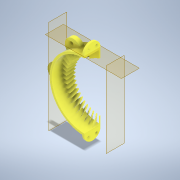
# Autodesk Inventor part: HalfShell.48.3.0
Saved by Autodesk Inventor 2021.2 (Build 252289000, 289)
## iProperties
Created: 2021-03-12
Part Number: HalfShell.48.3.0
Material: Generic
Document SubType Name: Modeling
Designer: Ryan
Density: 1 g/cm^3
Appearance: Smooth - Yellow
Author: Ryan
## iProperties of the stored document _3DPrint.ipt
Created: 2021-05-17
Part Number: _3DPrint
Material: Generic
Document SubType Name: Modeling
Designer: Ryan
Density: 1 g/cm^3
Appearance: Default
Author: Ryan
Autodesk Inventor part; units mm, degrees
ref_plane "XY Plane" through (0, 0, 0) normal (0, 0, 1) x (1, 0, 0)
sketch "Sketch1" plane through (0, 0, 0) normal (0, 0, 1) x (1, 0, 0)
  circle A0 centre (0, 0) radius 50.8
  circle A1 centre (0, 0) radius 53.975
  dimension "d0" = 101.6
  dimension "d1" = 107.95
  constraints: 2 centre point, 2 coincident
  measures "d0" diameter of A0
  measures "d1" diameter of A1
extrude "Extrusion1" add sketch "Sketch1" along normal blind 25.4
ref_plane "Work Plane1" through (35.56, 0, 0) normal (1, 0, 0) x (0, 1, 0)
ref_plane "Work Plane2" through (0, 53.975, 0) normal (0, 1, 0) x (-1, 0, 0)
sketch "Sketch3" plane through (0, 53.975, 0) normal (0, 1, 0) x (-1, 0, 0)
  line L0 (53.975, 0) -> (-53.975, 0) projected
  line L1 (3.175, 25.4) -> (-3.175, 25.4)
  line L2 (-3.175, 25.4) -> (-3.175, 0)
  line L3 (-3.175, 0) -> (3.175, 0)
  line L4 (3.175, 0) -> (3.175, 25.4)
  line L5 (3.175, 25.4) -> (-3.175, 0) construction
  line L6 (-3.175, 25.4) -> (3.175, 0) construction
  line L7 (53.975, 25.4) -> (-53.975, 25.4) projected
  point P0 (0, 0)
  point P1 (0, 12.7)
  point P2 (3.175, 0)
  dimension "d11" = 6.35
  dimension "d12" = 0
  constraints: 12 end point, 2 midpoint, 2 parallel, 1 horizontal, 1 perpendicular, 1 point on line
  measures "d11" distance of L3.end L2.end
  measures "d12" distance between parallel lines of L7 L1
extrude "Extrusion3" add sketch "Sketch3" along normal blind 12.7
fillet "Fillet1" radius 12.7 2 edges at (0, 66.675, 25.4) (0, 66.675, 0)
sketch "Sketch4" plane through (3.175, 53.975, 25.4) normal (1, 0, 0) x (0, 0, -1)
  circle A0 centre (6.35, 5.08) radius 1.5875
  line L0 (-5.08, 0) -> (30.48, 0) projected
  line L1 (0, 0) -> (0, -107.95) projected
  circle A1 centre (19.05, 5.08) radius 1.5875
  line L2 (25.4, 0) -> (25.4, -107.95) projected
  point P0 (25.4, -53.975)
  dimension "d16" = 3.175
  dimension "d17" = 5.08
  dimension "d40" = 6.35
  dimension "d41" = 3.175
  dimension "d42" = 6.35
  dimension "d43" = 5.08
  constraints: 2 centre point
  measures "d16" diameter of A0
  measures "d17" distance from line of L0 A0.centre
  measures "d40" horizontal distance of A0.centre L1.start
  measures "d41" diameter of A1
  measures "d42" horizontal distance of L2.start A1.centre
  measures "d43" distance from line of L0 A1.centre
extrude "Extrusion4" cut sketch "Sketch4" against normal blind 12.7
pattern_circular "Circular Pattern2" count 2 over 360 about axis through (0, 0, 0) along (0, 0, 1) of "Extrusion4", "Fillet1", "Extrusion3"
ref_plane "Work Plane3" through (-53.975, 0, 0) normal (1, 0, 0) x (0, 1, 0)
sketch "Sketch5" plane through (-53.975, 0, 0) normal (1, 0, 0) x (0, 1, 0)
  line L0 (-12.7, 9.525) -> (12.7, 9.525)
  line L1 (12.7, 9.525) -> (12.7, 15.875)
  line L2 (12.7, 15.875) -> (-12.7, 15.875)
  line L3 (-12.7, 15.875) -> (-12.7, 9.525)
  line L4 (-12.7, 9.525) -> (12.7, 15.875) construction
  line L5 (12.7, 9.525) -> (-12.7, 15.875) construction
  point P0 (0, 0)
  point P1 (0, 12.7)
  dimension "d24" = 25.4
  dimension "d25" = 6.35
  dimension "d26" = 12.7
  dimension "d27" = 0
  constraints: 12 end point, 2 midpoint, 2 parallel, 1 horizontal, 1 perpendicular
  measures "d24" distance of L2.end L1.end
  measures "d25" distance of L1.end L0.end
  measures "d26" distance of point (0, 12.7) point (0, 0)
  measures "d27" horizontal distance of point (0, 12.7) point (0, 0)
extrude "Extrusion5" add sketch "Sketch5" along normal blind 2.54
sketch "Sketch6" plane through (-53.975, 0, 0) normal (-1, 0, 0) x (0, 0, 1)
  line L0 (15.875, 0) -> (15.875, -12.7) projected
  line L1 (9.525, 12.7) -> (15.875, 12.7)
  line L2 (15.875, 12.7) -> (15.875, -12.7)
  line L3 (15.875, -12.7) -> (9.525, -12.7)
  line L4 (9.525, -12.7) -> (9.525, 12.7)
  line L5 (9.525, 12.7) -> (15.875, -12.7) construction
  line L6 (15.875, 12.7) -> (9.525, -12.7) construction
  point P0 (0, 0)
  point P1 (12.7, 0)
  constraints: 12 end point, 2 midpoint, 2 parallel, 1 horizontal, 1 perpendicular
extrude "Extrusion6" add sketch "Sketch6" along normal blind 12.7
fillet "Fillet2" radius 12.7 2 edges at (-66.675, 12.7, 12.7) (-66.675, -12.7, 12.7)
sketch "Sketch7" plane through (0, 0, 15.875) normal (0, 0, 1) x (1, 0, 0)
  circle A0 centre (-59.055, 0) radius 3.175
  line L0 (-53.975, 93.345) -> (-53.975, -93.345) projected
  point P0 (0, 0)
  dimension "d33" = 6.35
  dimension "d34" = 5.08
  constraints: 1 centre point
  measures "d33" diameter of A0
  measures "d34" distance from line of L0 A0.centre
extrude "Extrusion7" cut sketch "Sketch7" against normal blind 12.7
pattern_circular "Circular Pattern3" count 6 over 360 about axis through (0, 0, 0) along (0, 0, 1) of "Extrusion5", "Extrusion6", "Fillet2", "Extrusion7"
sketch "Sketch8" plane through (35.56, 0, 0) normal (1, 0, 0) x (0, 1, 0)
  line L0 (15.9757, 12.7) -> (24.5474, 12.7)
  line L1 (53.975, 25.4) -> (-53.975, 25.4) projected
  arc A0 (-0.5399, 1.5597) -> (5.5496, 11.9063) centre (-13.9916, 16.442) ccw
  arc A1 (0.6376, 0.3284) -> (5.5496, 11.9063) centre (-18.213, 15.157) ccw
  line L2 (53.975, 0) -> (-53.975, 0) projected
  arc A2 (-0.5399, 1.5597) -> (0.6376, 0.3284) centre (-0.0387, 0.8604) ccw
  dimension "d49" = 12.7
  dimension "d50" = 0.7937
  constraints: 6 point on circle, 3 centre point, 2 end point, 2 tangent, 1 horizontal
  measures "d49" distance between parallel lines of L1 L0
  measures "d50" distance from line of A0.end L0
extrude "Extrusion14" add sketch "Sketch8" along normal blind 16.51
pattern_circular "Circular Pattern9" count 48 over 360 about axis through (0, 0, 0) along (0, 0, 1) of "Extrusion14"
sketch "Sketch11" plane through (0, 0, 0) normal (0, 0, -1) x (-1, 0, 0)
  circle A0 centre (0, 0) radius 38.8938
  dimension "d84" = 77.7875
  constraints: 1 centre point, 1 coincident
  measures "d84" diameter of A0
extrude "Extrusion15" cut sketch "Sketch11" against normal through all draft 11.31
sketch "Sketch12" plane through (0, 0, 25.4) normal (0, 0, 1) x (1, 0, 0)
  line L0 (-3.175, 66.675) -> (3.175, 66.675) projected
  line L1 (0, 66.675) -> (72.4125, 66.675)
  line L2 (72.4125, 66.675) -> (72.4125, -76.6745)
  line L3 (72.4125, -76.6745) -> (0, -76.6745)
  line L4 (0, -76.6745) -> (0, 66.675)
  point P0 (0, 0)
  point P1 (3.175, 66.675)
  constraints: 8 end point, 2 parallel, 1 horizontal, 1 midpoint, 1 perpendicular
extrude "Extrusion16" cut sketch "Sketch12" against normal through all
sketch "Sketch13" plane through (0, 0, 25.4) normal (0, 0, 1) x (1, 0, 0)
  line L0 (-0.3508, 43.0001) -> (2.4324, 43.0001)
  line L1 (2.4324, 43.0001) -> (2.4324, 40.3013)
  line L2 (2.4324, 40.3013) -> (-0.3508, 40.3013)
  line L3 (-0.3508, 40.3013) -> (-0.3508, 43.0001)
  point P0 (0, 0)
  constraints: 8 end point, 2 parallel, 1 horizontal, 1 perpendicular
extrude "Extrusion17" cut sketch "Sketch13" against normal blind 20.32
body "Solid1"
